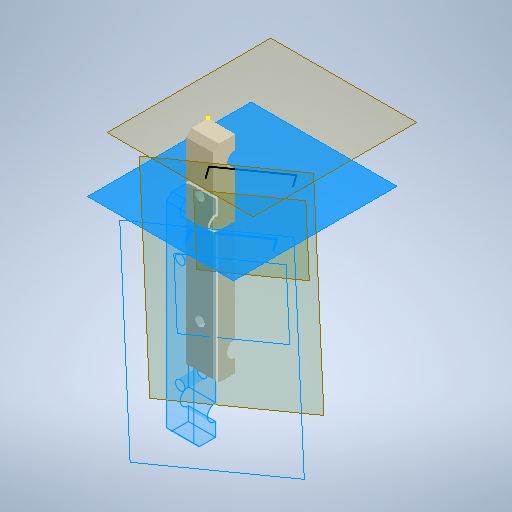
# Autodesk Inventor part: 6_2xclamp_main
Saved by Autodesk Inventor 2025.1 (Build 291241000, 241)
## iProperties
Created: 2024-10-31
Part Number: 6_2xclamp_main
Material: Ogólny
Document SubType Name: Modeling
Designer: PC
Density: 1 g/cm^3
Appearance: Domyślna
Author: PC
Autodesk Inventor part; units mm, degrees
ref_plane "YZ Plane" through (0, 0, 0) normal (1, 0, 0) x (0, 1, 0)
ref_plane "XZ Plane" through (0, 0, 0) normal (0, 1, 0) x (-1, 0, 0)
ref_plane "XY Plane" through (0, 0, 0) normal (0, 0, 1) x (1, 0, 0)
sketch "Szkic1" plane through (0, 0, 0) normal (1, 0, 0) x (0, 1, 0)
  circle A0 centre (0, 0) radius 3 construction
  circle A1 centre (60, 0) radius 3 construction
  arc A2 (63, 0) -> (57, 0) centre (60, 0) ccw
  arc A3 (3, 0) -> (-3, 0) centre (0, 0) ccw
  line L0 (68, 0) -> (68, 8)
  line L1 (68, 8) -> (-8, 8)
  line L2 (-8, 8) -> (-8, 0)
  line L3 (63, 0) -> (68, 0)
  line L4 (-8, 0) -> (-3, 0)
  line L5 (3, 0) -> (57, 0)
  point P0 (-5.5, 0)
  dimension "d0" = 6
  dimension "d1" = 6
  dimension "d2" = 60
  dimension "d3" = 6
  dimension "d4" = 5
  dimension "d5" = 8
  constraints: 12 end point, 4 centre point, 4 parallel, 4 point on circle, 3 coincident, 3 horizontal, 3 perpendicular, 1 collinear, 1 concentric, 1 midpoint
  measures "d0" diameter of A0
  measures "d1" diameter of A1
  measures "d2" distance of point (0, 0) A1.centre
  measures "d3" diameter of A3
  measures "d4" distance of L3.start L0.start
  measures "d5" distance from line of point (-5.5, 0) L1
extrude "Wyciągnięcie proste1" add sketch "Szkic1" along normal blind 10
sketch "Szkic2" plane through (0, 3, 0) normal (0, 0, -1) x (-1, 0, 0)
  line L0 (0, 65) -> (-10, 65) construction
  line L1 (-5, 65) -> (-5, -11.1641) construction
  line L2 (-10, 65) -> (-10, -11) construction
  line L3 (-10, 27) -> (0, 27) construction
  line L4 (0, 65) -> (0, -11) construction
  circle A0 centre (-5, 47) radius 1.75
  circle A1 centre (-5, 7) radius 1.75
  circle A2 centre (-5, 37) radius 1.75
  circle A3 centre (-5, 17) radius 1.75
  point P0 (0, -3)
  dimension "d8" = 3.5
  dimension "d9" = 20
  dimension "d15" = 3.5
  dimension "d16" = 10
  constraints: 4 centre point, 4 end point, 3 midpoint, 2 point on line, 2 symmetric about line, 1 vertical, 2 other
  measures "d8" diameter of A0
  measures "d9" distance from line of L3 A0.centre
  measures "d15" diameter of A2
  measures "d16" distance from line of L3 A2.centre
extrude "Wyciągnięcie proste2" cut sketch "Szkic2" against normal up to next contours A0 | A1
chamfer "Faza1" distance 2 angle 45 2 edges at (5, 68, 8) (5, -8, 8)
ref_plane "Płaszczyzna konstrukcyjna1" through (5, 68, 6) normal (0, 1, 0) x (1, 0, 0)
sketch "Szkic3" plane through (5, 68, 6) normal (0, 1, 0) x (1, 0, 0)
  point P0 (-5, 6)
sketch "Szkic4" plane through (5, 68, 6) normal (0, 1, 0) x (1, 0, 0)
  line L0 (29.238, 4.1877) -> (10.4797, -9.1212)
  line L1 (11.1628, -10.084) -> (10.4797, -9.1212)
  line L2 (13.5481, -13.4459) -> (11.1628, -10.084)
  line L3 (29.9211, 3.2248) -> (29.238, 4.1877)
  line L4 (29.9211, 3.2248) -> (32.3064, -0.1371)
  point P0 (-5, 6)
  constraints: 10 end point, 11 other
ref_plane "Płaszczyzna konstrukcyjna2" through (17.8649, 60.2933, 18.4831) normal (-0.569277, 0.1792222, -0.8023734) x (0.1037062, 0.9838086, 0.1461698)
ref_plane "Płaszczyzna konstrukcyjna3" through (26.0515, 48.9795, 10.1477) normal (-0.569277, 0.1792222, -0.8023734) x (0.8155788, 0, -0.5786461)
sketch "Szkic5" plane through (26.0515, 48.9795, 10.1477) normal (-0.569277, 0.1792222, -0.8023734) x (0.8155788, 0, -0.5786461)
  line L0 (11.5, -11.5) -> (11.5, 11.5) construction
  line L1 (11.5, 11.5) -> (-11.5, 11.5) construction
  line L2 (-11.5, 11.5) -> (-11.5, -11.5) construction
  line L3 (-11.5, -11.5) -> (11.5, -11.5) construction
  line L4 (-11.5, 11.5) -> (18.547, 11.5)
  line L5 (18.547, 11.5) -> (18.547, -17.121)
  line L6 (18.547, -17.121) -> (-11.5, -17.121)
  line L7 (-11.5, -17.121) -> (-11.5, 11.5)
  circle A0 centre (14.589, 7.796) radius 1.45
  line L8 (18.547, -17.121) -> (-11.5, 11.5) construction
  circle A1 centre (-6.5329, -14.3782) radius 1.45
  point P0 (-15.3751, 52.3715)
  dimension "d17" = 30.047
  dimension "d18" = 2.9
  dimension "d19" = 3.704
  dimension "d20" = 3.958
  dimension "d21" = 28.621
  constraints: 18 end point, 3 horizontal, 2 centre point, 2 parallel, 2 vertical, 1 perpendicular, 1 symmetric about line, 5 other
  measures "d17" distance of L1.end L4.end
  measures "d18" diameter of A0
  measures "d19" distance from line of L4 A0.centre
  measures "d20" distance from line of L5 A0.centre
  measures "d21" distance from line of L4 L5.end
extrude "Wyciągnięcie proste3" [suppressed]
sketch "Szkic6" plane through (18.5909, 67.18, 19.5063) normal (0.1037062, 0.9838086, 0.1461698) x (0.8155788, 0, -0.5786461)
  line L0 (0, 0) -> (30, 0) projected
  line L1 (30, 0) -> (30, 4) projected
  line L2 (0, 4) -> (30, 4) projected
  line L3 (0, 0) -> (0, 4) projected
  line L4 (2, 7) -> (26.5831, 7)
  line L5 (26.5831, 7) -> (26.5831, 10)
  line L6 (26.5831, 10) -> (0, 10)
  line L7 (0, 10) -> (0, 4)
  arc A0 (2, 7) -> (2, 4) centre (2, 5.5) ccw
  point P0 (-3.8751, 14.1945)
  dimension "d24" = 3
  dimension "d25" = 2.042
  dimension "d26" = 3.062
  constraints: 8 end point, 3 perpendicular, 2 point on circle, 2 tangent, 1 centre point, 1 point on line
  measures "d24" distance of L4.end L5.end
extrude "Wyciągnięcie proste4" [suppressed]
sketch "Szkic7" plane through (34.5787, 68.9722, -3.8997) normal (-0.569277, 0.1792222, -0.8023734) x (-0.8155788, 0, 0.5786461)
  line L0 (26.5831, -27.9454) -> (26.3218, -30) projected
  line L1 (26.5831, 0) -> (26.5831, -27.9454) projected
  line L2 (0, 0) -> (26.5831, 0) projected
  line L3 (0, 0) -> (0, -30) projected
  line L4 (0, -30) -> (26.3218, -30) projected
  line L5 (0, -20) -> (0, -10)
  line L6 (0, 0) -> (0, -30) projected
  line L7 (26.5831, 0) -> (26.5831, -26.8739)
  circle A0 centre (4, -15) radius 1.45
  line L8 (26.5831, 0) -> (26.5831, -30)
  line L9 (26.5831, -30) -> (21.5831, -30)
  line L10 (-3.4169, -30) -> (24.5831, -30) projected
  line L11 (21.5831, -30) -> (0, -20)
  line L12 (0, -10) -> (21.5831, 0)
  line L13 (26.5831, 0) -> (21.5831, 0)
  line L14 (21.5831, -30) -> (26.5831, -30)
  point P0 (30.4582, -70.8715)
  point P1 (0, -15)
  point P2 (0, -10)
  point P3 (21.5831, -30)
  dimension "d29" = 11.638
  dimension "d32" = 2.9
  dimension "d33" = 6.646
  dimension "d34" = 3.439
  constraints: 16 end point, 5 point on line, 2 collinear, 1 centre point, 1 equal length, 1 midpoint, 1 parallel, 1 vertical, 1 vertical alignment
  measures "d32" diameter of A0
extrude "Wyciągnięcie proste5" [suppressed]
sketch "Szkic11" plane through (10, 0, 0) normal (1, 0, 0) x (0, 0, -1)
  line L0 (6.8231, 49.296) -> (-4.2042, 39.4579) projected
  line L1 (-4.2042, 39.4579) -> (-6.9463, 39.4579) projected
  line L2 (-7.3978, 41.4793) -> (-6.9463, 39.4579) projected
  line L3 (-11.4825, 68.9722) -> (-7.3978, 41.4793) projected
  line L4 (-8.5893, 68.9722) -> (-11.4825, 68.9722) projected
  line L5 (-8.5893, 68.9722) -> (5.3614, 59.1341) projected
  line L6 (5.3614, 59.1341) -> (6.8231, 49.296) projected
  ellipse E0 centre (3.7776, 54.2151) end of major axis (4.0937, 52.7999) minor radius 0.8255 projected
  line L7 (0, 3) -> (0, 57) projected
  line L8 (-8, 66) -> (-8, -6) projected
  line L9 (0, 43.2088) -> (0, 62.915)
  line L10 (0, 62.915) -> (-6.5007, 67.4993)
  line L11 (-6.5007, 67.4993) -> (-8, 66)
  line L12 (-8, 66) -> (-8, 45.5327)
  point P0 (0, 0)
  point P1 (0, 0)
  point P2 (0, 0)
  point P3 (0, 0)
  point P4 (0, 0)
  constraints: 8 end point, 6 point on line, 2 coincident, 1 vertical
extrude "Wyciągnięcie proste8" [suppressed]
sketch "Szkic8" plane through (10, 0, 0) normal (1, 0, 0) x (0, 0, -1)
  line L0 (-2.1469, 67.18) -> (2.2382, 37.6657) projected
  line L1 (2.2382, 37.6657) -> (5.4477, 38.3826) projected
  line L2 (1.0626, 67.8969) -> (5.4477, 38.3826) projected
  line L3 (-2.1469, 67.18) -> (1.0626, 67.8969) projected
  line L4 (1, 2.8284) -> (1, 57.1716)
  line L5 (5.3614, 59.1341) -> (6.8231, 49.296) projected
  arc A0 (0, 63) -> (0, 57) centre (0, 60) ccw projected
  line L6 (9.8159, 60) -> (9.8159, 68.4413)
  line L7 (9.8159, 68.4413) -> (-3.5, 68.4413)
  line L8 (-3.5, 68.4413) -> (-3.5, 60)
  line L9 (0, 56.5) -> (9.8159, 56.5)
  line L10 (9.8159, 56.5) -> (9.8159, 60)
  arc A1 (-3.5, 60) -> (0, 56.5) centre (0, 60) ccw
  point P0 (0, 0)
  dimension "d42" = 3.5
  constraints: 12 end point, 2 point on circle, 1 centre point, 1 coincident, 1 collinear, 1 horizontal, 1 parallel, 1 tangent, 1 vertical, 2 other
  measures "d42" radius of A1
extrude "Wyciągnięcie proste6" [suppressed]
sketch "Szkic12" plane through (17.091, 68.1657, 13.9359) normal (0.1037062, 0.9838086, 0.1461698) x (0.8155788, 0, -0.5786461)
  line L0 (20.9791, -1.5) -> (18.9515, -1.5) projected
  line L1 (26.5257, -5.5) -> (20.9791, -1.5) projected
  line L2 (24.6821, -5.5) -> (26.5257, -5.5) projected
  line L3 (18.9515, -1.5) -> (24.6821, -5.5) projected
  line L4 (28, -5.5) -> (-2, -5.5) projected
  line L5 (18.9515, -1.5) -> (28, -1.5)
  line L6 (28, -1.5) -> (28, -5.5)
  line L7 (28, -5.5) -> (18.9515, -5.5)
  line L8 (18.9515, -5.5) -> (18.9515, -1.5)
  point P0 (-5.8751, 8.6945)
  point P1 (18.9515, -5.5)
  constraints: 8 end point, 2 parallel, 1 horizontal, 1 perpendicular
extrude "Wyciągnięcie proste9" [suppressed]
sketch "Szkic13" plane through (0, 0, 0) normal (-1, 0, 0) x (0, 0, 1)
  line L0 (6.5007, 67.4993) -> (8, 66) projected
  line L1 (8, 66) -> (8, 45.5327) projected
  line L2 (11.4825, 68.9722) -> (8, 45.5327) projected
  line L3 (8.5893, 68.9722) -> (11.4825, 68.9722) projected
  line L4 (8.5893, 68.9722) -> (6.5007, 67.4993) projected
  line L5 (63.0199, 65.5599) -> (-3.0201, 65.5599)
  line L6 (15.1212, 37.6657) -> (19.5063, 67.18) projected
  line L7 (19.5063, 67.18) -> (11.4825, 68.9722) projected
  line L8 (11.4825, 68.9722) -> (8, 45.5327) projected
  line L9 (8, 45.5327) -> (7.3978, 41.4793) projected
  line L10 (7.3978, 39.3909) -> (7.3978, 41.4793) projected
  line L11 (15.1212, 37.6657) -> (7.3978, 39.3909) projected
  line L12 (8, -6) -> (6, -8) projected
  line L13 (8, 66) -> (8, -6) projected
  line L14 (6, 68) -> (8, 66) projected
  line L15 (0, 68) -> (6, 68) projected
  line L16 (0, 63) -> (0, 68) projected
  arc A0 (0, 57) -> (0, 63) centre (0, 60) ccw projected
  line L17 (0, 3) -> (0, 57) projected
  arc A1 (0, -3) -> (0, 3) centre (0, 0) ccw projected
  line L18 (0, -8) -> (0, -3) projected
  line L19 (6, -8) -> (0, -8) projected
  line L20 (8, 66) -> (8, -6) projected
  line L21 (8, 39.2563) -> (0, 39.2563)
  line L22 (0, 3) -> (0, 57) projected
  point P0 (8, 39.2563)
  constraints: 4 end point, 3 point on line, 2 horizontal, 2 other
extrude "Wyciągnięcie proste10" [suppressed]
sketch "Szkic14" plane through (10.4273, 45.5327, 8) normal (0.8155788, 0, -0.5786461) x (-0.5786461, 0, -0.8155788)
  point P0 (12.5583, -45.5327)
sketch "Szkic15" plane through (10.4273, 45.5327, 8) normal (0.8155788, 0, -0.5786461) x (-0.5786461, 0, -0.8155788)
  line L0 (-4.27, 23.4395) -> (0, 0) projected
  line L1 (0, 20.4673) -> (0, 0) projected
  line L2 (1.8383, 21.9666) -> (0, 20.4673) projected
  line L3 (1.8383, 21.9666) -> (-0.7226, 23.4395) projected
  line L4 (-0.7226, 23.4395) -> (-4.27, 23.4395) projected
  point P0 (12.5583, -45.5327)
sketch "Szkic16" plane through (0, 68, 0) normal (0, 1, 0) x (1, 0, 0)
  line L0 (0, 0) -> (43.9824, 0)
  line L1 (43.9824, 0) -> (43.9824, -26.4065)
  line L2 (43.9824, -26.4065) -> (0, -26.4065)
  line L3 (0, -26.4065) -> (0, 0)
  constraints: 8 end point, 2 parallel, 1 horizontal, 1 perpendicular
extrude "Wyciągnięcie proste11" [suppressed]
sketch "Szkic17" plane through (0, 67, 0) normal (0, 1, 0) x (1, 0, 0)
  point P0 (0, 0)
sketch "Szkic18" plane through (0, 67, 0) normal (0, 1, 0) x (1, 0, 0)
  line L0 (20.2969, -5.7927) -> (21.0993, -8.9622) projected
  line L1 (20.2969, -5.7927) -> (11.6216, -12.236)
  line L2 (11.6216, -12.236) -> (8.0042, -6.3815)
  line L3 (8.0042, -6.3815) -> (20.2969, -5.7927)
  point P0 (0, 0)
  constraints: 6 end point
extrude "Wyciągnięcie proste12" [suppressed]
sketch "Szkic19" plane through (0, 67, 0) normal (0, 1, 0) x (1, 0, 0)
  point P0 (0, 0)
